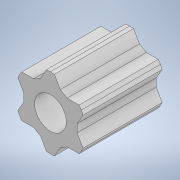
# Autodesk Inventor part: Część5
Saved by Autodesk Inventor 2020 (Build 240168000, 168)
## iProperties
Created: 2021-10-14
Part Number: Część5
Material: Ogólny
Document SubType Name: Modeling
Designer: Komputer
Density: 1 g/cm^3
Appearance: Domyślna
Author: Komputer
Autodesk Inventor part; units mm, degrees
ref_plane "YZ Plane" through (0, 0, 0) normal (1, 0, 0) x (0, 1, 0)
ref_plane "XZ Plane" through (0, 0, 0) normal (0, 1, 0) x (-1, 0, 0)
ref_plane "XY Plane" through (0, 0, 0) normal (0, 0, 1) x (1, 0, 0)
sketch "Szkic1" plane through (0, 0, 0) normal (0, 0, 1) x (1, 0, 0)
  line L0 (-0.0008, 4.5) -> (-0.5, 4.4721)
  line L1 (-0.0008, 4.5) -> (0.5, 4.4721)
  line L2 (0.5, 4.4721) -> (1.6267, 2.5207)
  line L3 (0.5, 4.4721) -> (2.7533, 4.4721) construction
  line L4 (-0.0008, 4.5) -> (-0.5, 4.4721)
  line L5 (-0.5, 4.4721) -> (-1.6255, 2.5215)
  line L6 (-4.4721, 0.5) -> (-2.5207, 1.6267)
  line L7 (-4.5, -0.0008) -> (-4.4721, 0.5)
  line L8 (-4.5, -0.0008) -> (-4.4721, -0.5)
  line L9 (-4.4721, -0.5) -> (-2.5215, -1.6255)
  line L10 (-0.5, -4.4721) -> (-1.6267, -2.5207)
  line L11 (0.0008, -4.5) -> (-0.5, -4.4721)
  line L12 (0.0008, -4.5) -> (0.5, -4.4721)
  line L13 (0.5, -4.4721) -> (1.6255, -2.5215)
  line L14 (4.4721, -0.5) -> (2.5207, -1.6267)
  line L15 (4.5, 0.0008) -> (4.4721, -0.5)
  line L16 (4.5, 0.0008) -> (4.4721, 0.5)
  line L17 (4.4721, 0.5) -> (2.5215, 1.6255)
  line L18 (-4.4721, -0.5) -> (-3.1729, -1.2496)
  circle A0 centre (0, 0) radius 3.4101
  line L19 (-4.123, 1.8031) -> (-2.9964, -0.147)
  line L20 (-3.8975, 2.2493) -> (-4.123, 1.8031)
  line L21 (-3.8975, 2.2493) -> (-3.623, 2.6691)
  line L22 (-3.623, 2.6691) -> (-1.3697, 2.6691)
  line L23 (-3.623, -2.6691) -> (-1.3709, -2.6685)
  line L24 (-3.8967, -2.2507) -> (-3.623, -2.6691)
  line L25 (-3.8967, -2.2507) -> (-4.123, -1.8031)
  line L26 (-4.123, -1.8031) -> (-2.9963, 0.1484)
  line L27 (0.5, -4.4721) -> (1.6255, -2.5215)
  line L28 (0.0008, -4.5) -> (0.5, -4.4721)
  line L29 (0.0008, -4.5) -> (-0.5, -4.4721)
  line L30 (-0.5, -4.4721) -> (-1.6267, -2.5207)
  line L31 (4.123, -1.8031) -> (2.9964, 0.147)
  line L32 (3.8975, -2.2493) -> (4.123, -1.8031)
  line L33 (3.8975, -2.2493) -> (3.623, -2.6691)
  line L34 (3.623, -2.6691) -> (1.3697, -2.6691)
  line L35 (3.623, 2.6691) -> (1.3709, 2.6685)
  line L36 (3.8967, 2.2507) -> (3.623, 2.6691)
  line L37 (3.8967, 2.2507) -> (4.123, 1.8031)
  line L38 (4.123, 1.8031) -> (2.9963, -0.1484)
  line L39 (-2.1225, 2.6691) -> (-1.2496, 3.1729)
  line L40 (1.2503, 3.1726) -> (2.123, 2.6687)
  line L41 (3.3727, 0.5036) -> (3.3726, -0.5042)
  line L42 (2.1225, -2.6691) -> (1.2496, -3.1729)
  line L43 (-1.2503, -3.1726) -> (-2.123, -2.6687)
  line L44 (-3.3727, -0.5036) -> (-3.3726, 0.5042)
  point P0 (-1.2503, -3.1726)
  point P1 (1.2496, -3.1729)
  point P2 (3.1726, -1.2503)
  point P3 (3.1729, 1.2496)
  point P4 (1.2503, 3.1726)
  point P5 (-1.2496, 3.1729)
  point P6 (-3.1726, 1.2503)
  point P7 (-3.6459, -0.9767)
  point P8 (-1.2503, -3.1726)
  point P9 (1.2496, -3.1729)
  dimension "d2" = 0.5
  dimension "d3" = 60
  dimension "d8" = 360
  dimension "d12" = 1.5
  dimension "d15" = 360
  constraints: 90 end point, 13 point on line, 1 equal length, 1 horizontal, 107 other
  measures "d2" distance of L0.start L0.end
  measures "d3" angle of L2 L3
  measures "d12" distance of L8.end L18.end
extrude "Wyciągnięcie proste2" add sketch "Szkic1" along normal blind 10 contours L1 L2 A0 L5 L0 | A0 L2 L35 L38 L31 L34 L13 L10 L23 L26 L19 L22 L5 | L5 L22 L39 | L40 L35 L2 | A0 L6 L19 L20 L21 L22 | L35 L36 L37 L38 L17 A0 | A0 L19 L6 | L17 L38 A0 | L19 L26 L44 | L41 L31 L38 | A0 L9 L26 | L31 L14 A0 | A0 L23 L24 L25 L26 L9 | L14 L31 L32 L33 L34 A0 | L23 L10 L43 | L42 L13 L34 | A0 L13 L12 L11 L10
sketch "Szkic2" plane through (0, 0, 0) normal (0, 0, -1) x (-1, 0, 0)
  circle A0 centre (0, 0) radius 2
  dimension "d19" = 4
  constraints: 1 centre point, 1 coincident
  measures "d19" diameter of A0
sketch "Szkic3" plane through (0, 0, 0) normal (0, 0, -1) x (-1, 0, 0)
  point P0 (0, 0)
extrude "Wyciągnięcie proste3" cut sketch "Szkic2" against normal blind 10
